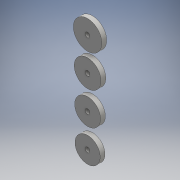
# Autodesk Inventor part: BearingSilicone_Spacer_3mm
Saved by Autodesk Inventor 2016 (Build 200138000, 138)
## iProperties
Created: 2015-12-22
Part Number: BearingSilicone_Spacer_3mm
Material: Generic
Document SubType Name: Modeling
Designer: momem
Density: 1 g/cm^3
Appearance: Default
Author: momem
Autodesk Inventor part; units mm, degrees
ref_plane "YZ Plane" through (0, 0, 0) normal (1, 0, 0) x (0, 1, 0)
ref_plane "XZ Plane" through (0, 0, 0) normal (0, 1, 0) x (-1, 0, 0)
ref_plane "XY Plane" through (0, 0, 0) normal (0, 0, 1) x (1, 0, 0)
sketch "Sketch1" plane through (0, 0, 0) normal (0, 1, 0) x (-1, 0, 0)
  circle A0 centre (0, 0) radius 1.5875
  circle A1 centre (0, 0) radius 9.45
  circle A2 centre (0, -22) radius 1.5875
  circle A3 centre (0, -22) radius 8.9
  circle A4 centre (0, -44) radius 1.5875
  circle A5 centre (0, -44) radius 8.57
  circle A6 centre (0, -66) radius 1.5875
  circle A7 centre (0, -66) radius 8.35
  dimension "d19" = 3.175
  dimension "d20" = 18.9
  dimension "d21" = 3.175
  dimension "d22" = 17.8
  dimension "d24" = 3.175
  dimension "d25" = 17.14
  dimension "d27" = 3.175
  dimension "d28" = 16.7
  dimension "d30" = 22
  dimension "d31" = 22
  dimension "d32" = 22
  constraints: 8 centre point, 5 coincident, 3 vertical alignment
  measures "d19" diameter of A0
  measures "d20" diameter of A1
  measures "d21" diameter of A2
  measures "d22" diameter of A3
  measures "d24" diameter of A4
  measures "d25" diameter of A5
  measures "d27" diameter of A6
  measures "d28" diameter of A7
  measures "d30" distance of A2.centre point (0, 0)
  measures "d31" distance of A4.centre A2.centre
  measures "d32" distance of A6.centre A4.centre
extrude "Extrusion1" add sketch "Sketch1" along normal blind 3.195
equation "\"d33\" = 0.5 * WoodThickness"
equation "\"WoodThickness\" = 6.39"
body "Solid1"
